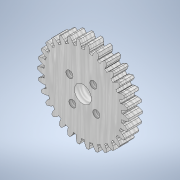
# Autodesk Inventor part: m1歯数30ギア5t
Saved by Autodesk Inventor 2020.2 (Build 242310000, 310)
## iProperties
Created: 2020-02-29
Part Number: m1歯数30ギア5t
Material: アルミニウム 7075
Document SubType Name: Modeling
Designer: aoyam
Density: 2.81 g/cm^3
Appearance: サテン - ブラシ仕上げ 重厚
Author: aoyam
Autodesk Inventor part; units mm, degrees
ref_plane "YZ Plane" through (0, 0, 0) normal (1, 0, 0) x (0, 1, 0)
ref_plane "XZ Plane" through (0, 0, 0) normal (0, 1, 0) x (-1, 0, 0)
ref_plane "XY Plane" through (0, 0, 0) normal (0, 0, 1) x (1, 0, 0)
sketch "スケッチ1" plane through (0, 0, 0) normal (0, 0, 1) x (1, 0, 0)
  arc A0 (3.2208, 16.1154) -> (3.1922, 15.9239) centre (4.5004, 15.8268) ccw
  arc A1 (3.406, 16.7122) -> (3.2208, 16.1154) centre (6.7386, 15.3507) ccw
  arc A2 (3.9698, 17.7851) -> (3.406, 16.7122) centre (9.1484, 14.3793) ccw
  arc A3 (2.1366, 15.9239) -> (2.108, 16.1154) centre (0.8284, 15.8268) ccw
  arc A4 (2.108, 16.1154) -> (1.9228, 16.7122) centre (-1.4098, 15.3507) ccw
  arc A5 (1.9228, 16.7122) -> (1.359, 17.7851) centre (-3.8196, 14.3793) ccw
  arc A6 (3.1793, 15.5788) -> (2.1495, 15.5788) centre (2.6644, 1.8384) ccw
  arc A7 (1.359, 17.7851) -> (0.6257, 17.708) centre (2.6644, 1.8384) ccw
  line L0 (3.1793, 15.5788) -> (3.1922, 15.9239)
  line L1 (2.1495, 15.5788) -> (2.1366, 15.9239)
  arc A8 (0.2403, 15.9191) -> (0.2521, 15.7259) centre (1.5519, 15.9028) ccw
  line L2 (0.3113, 15.3856) -> (0.2521, 15.7259)
  arc A9 (0.2973, 16.5413) -> (0.2403, 15.9191) centre (3.8402, 15.9025) ccw
  arc A10 (0.6257, 17.708) -> (0.2973, 16.5413) centre (6.3993, 15.4534) ccw
  arc A11 (0.3113, 15.3856) -> (-0.696, 15.1715) centre (2.6644, 1.8384) ccw
  line L3 (-0.696, 15.1715) -> (-0.7804, 15.5064)
  arc A12 (-0.7804, 15.5064) -> (-0.8482, 15.6877) centre (-2.0398, 15.1394) ccw
  arc A13 (-1.1534, 16.233) -> (-1.9279, 17.1652) centre (-6.2853, 12.7572) ccw
  arc A14 (-1.9279, 17.1652) -> (-2.6292, 16.9374) centre (2.6644, 1.8384) ccw
  arc A15 (-0.8482, 15.6877) -> (-1.1534, 16.233) centre (-4.1301, 14.2084) ccw
  arc A16 (-2.6343, 15.1074) -> (-2.5825, 14.9209) centre (-1.3479, 15.3642) ccw
  line L4 (-2.4539, 14.6003) -> (-2.5825, 14.9209)
  arc A17 (-2.7078, 15.7279) -> (-2.6343, 15.1074) centre (0.8904, 15.8397) ccw
  arc A18 (-2.6292, 16.9374) -> (-2.7078, 15.7279) centre (3.487, 15.9324) ccw
  arc A19 (-2.4539, 14.6003) -> (-3.3947, 14.1814) centre (2.6644, 1.8384) ccw
  line L5 (-3.3947, 14.1814) -> (-3.5469, 14.4915)
  arc A20 (-3.5469, 14.4915) -> (-3.6508, 14.6548) centre (-4.7024, 13.8707) ccw
  arc A21 (-4.0628, 15.1246) -> (-5.0142, 15.8755) centre (-8.3599, 10.6578) ccw
  arc A22 (-5.0142, 15.8755) -> (-5.6528, 15.5068) centre (2.6644, 1.8384) ccw
  arc A23 (-3.6508, 14.6548) -> (-4.0628, 15.1246) centre (-6.5535, 12.5254) ccw
  arc A24 (-5.2773, 13.7158) -> (-5.1878, 13.5441) centre (-4.0724, 14.2344) ccw
  line L6 (-4.9954, 13.2573) -> (-5.1878, 13.5441)
  arc A25 (-5.4782, 14.3074) -> (-5.2773, 13.7158) centre (-1.9819, 15.1649) ccw
  arc A26 (-5.6528, 15.5068) -> (-5.4782, 14.3074) centre (0.5387, 15.7954) ccw
  arc A27 (-4.9954, 13.2573) -> (-5.8285, 12.652) centre (2.6644, 1.8384) ccw
  line L7 (-5.8285, 12.652) -> (-6.0419, 12.9236)
  arc A28 (-6.0419, 12.9236) -> (-6.1775, 13.0617) centre (-7.0431, 12.0761) ccw
  arc A29 (-6.6781, 13.4356) -> (-7.7649, 13.9723) centre (-9.9526, 8.173) ccw
  arc A30 (-7.7649, 13.9723) -> (-8.3128, 13.4789) centre (2.6644, 1.8384) ccw
  arc A31 (-6.1775, 13.0617) -> (-6.6781, 13.4356) centre (-8.574, 10.3754) ccw
  arc A32 (-7.5732, 11.8051) -> (-7.45, 11.6557) centre (-6.5025, 12.5629) ccw
  line L8 (-7.2021, 11.4152) -> (-7.45, 11.6557)
  arc A33 (-7.8927, 12.342) -> (-7.5732, 11.8051) centre (-4.651, 13.9076) ccw
  arc A34 (-8.3128, 13.4789) -> (-7.8927, 12.342) centre (-2.3167, 15.0485) ccw
  arc A35 (-7.2021, 11.4152) -> (-7.8912, 10.6499) centre (2.6644, 1.8384) ccw
  line L9 (-7.8912, 10.6499) -> (-8.1564, 10.8712)
  arc A36 (-8.1564, 10.8712) -> (-8.3177, 10.9781) centre (-8.9595, 9.8341) ccw
  arc A37 (-8.8852, 11.2398) -> (-10.0597, 11.5388) centre (-10.9939, 5.4114) ccw
  arc A38 (-10.0597, 11.5388) -> (-10.4931, 10.9422) centre (2.6644, 1.8384) ccw
  arc A39 (-8.3177, 10.9781) -> (-8.8852, 11.2398) centre (-10.1034, 7.8522) ccw
  arc A40 (-9.4216, 9.4587) -> (-9.2701, 9.3383) centre (-8.5319, 10.4226) ccw
  line L10 (-8.9777, 9.1545) -> (-9.2701, 9.3383)
  arc A41 (-9.8458, 9.9175) -> (-9.4216, 9.4587) centre (-7.0005, 12.1229) ccw
  arc A42 (-10.4931, 10.9422) -> (-9.8458, 9.9175) centre (-4.9544, 13.7242) ccw
  arc A43 (-8.9777, 9.1545) -> (-9.4925, 8.2627) centre (2.6644, 1.8384) ccw
  line L11 (-9.4925, 8.2627) -> (-9.7979, 8.4241)
  arc A44 (-9.7979, 8.4241) -> (-9.978, 8.4951) centre (-10.3679, 7.2426) ccw
  arc A45 (-10.5874, 8.6331) -> (-11.7985, 8.6813) centre (-11.4383, 2.4936) ccw
  arc A46 (-11.7985, 8.6813) -> (-12.0984, 8.0077) centre (2.6644, 1.8384) ccw
  arc A47 (-9.978, 8.4951) -> (-10.5874, 8.6331) centre (-11.0747, 5.0662) ccw
  arc A48 (-10.7419, 6.7794) -> (-10.5686, 6.6931) centre (-10.072, 7.9072) ccw
  line L12 (-10.2443, 6.5741) -> (-10.5686, 6.6931)
  arc A49 (-11.2522, 7.14) -> (-10.7419, 6.7794) centre (-8.9276, 9.8887) ccw
  arc A50 (-12.0984, 8.0077) -> (-11.2522, 7.14) centre (-7.2591, 11.8804) ccw
  arc A51 (-10.2443, 6.5741) -> (-10.5626, 5.5947) centre (2.6644, 1.8384) ccw
  line L13 (-10.5626, 5.5947) -> (-10.8948, 5.6891)
  arc A52 (-10.8948, 5.6891) -> (-11.0857, 5.7211) centre (-11.2067, 4.4149) ccw
  arc A53 (-11.7105, 5.7294) -> (-12.9052, 5.5247) centre (-11.2664, -0.4529) ccw
  arc A54 (-12.9052, 5.5247) -> (-13.0585, 4.8035) centre (2.6644, 1.8384) ccw
  arc A55 (-11.0857, 5.7211) -> (-11.7105, 5.7294) centre (-11.4456, 2.1392) ccw
  arc A56 (-11.4762, 3.8841) -> (-11.2888, 3.8357) centre (-11.0554, 5.1265) ccw
  line L14 (-10.9469, 3.7868) -> (-11.2888, 3.8357)
  arc A57 (-12.0503, 4.1307) -> (-11.4762, 3.8841) centre (-10.348, 7.3027) ccw
  arc A58 (-13.0585, 4.8035) -> (-12.0503, 4.1307) centre (-9.13, 9.5978) ccw
  arc A59 (-10.9469, 3.7868) -> (-11.0545, 2.7626) centre (2.6644, 1.8384) ccw
  line L15 (-11.0545, 2.7626) -> (-11.3991, 2.7858)
  arc A60 (-11.3991, 2.7858) -> (-11.5925, 2.7775) centre (-11.4392, 1.4747) ccw
  arc A61 (-12.2054, 2.6556) -> (-13.3314, 2.2071) centre (-10.4856, -3.2992) ccw
  arc A62 (-13.3314, 2.2071) -> (-13.3314, 1.4698) centre (2.6644, 1.8384) ccw
  arc A63 (-11.5925, 2.7775) -> (-12.2054, 2.6556) centre (-11.1998, -0.801) ccw
  arc A64 (-11.5925, 0.8994) -> (-11.3991, 0.891) centre (-11.4392, 2.2022) ccw
  line L16 (-11.0545, 0.9142) -> (-11.3991, 0.891)
  arc A65 (-12.2054, 1.0212) -> (-11.5925, 0.8994) centre (-11.1998, 4.4779) ccw
  arc A66 (-13.3314, 1.4698) -> (-12.2054, 1.0212) centre (-10.4856, 6.976) ccw
  arc A67 (-11.0545, 0.9142) -> (-10.9469, -0.1099) centre (2.6644, 1.8384) ccw
  line L17 (-10.9469, -0.1099) -> (-11.2888, -0.1588)
  arc A68 (-11.2888, -0.1588) -> (-11.4762, -0.2072) centre (-11.0554, -1.4497) ccw
  arc A69 (-12.0503, -0.4538) -> (-13.0585, -1.1267) centre (-9.13, -5.9209) ccw
  arc A70 (-13.0585, -1.1267) -> (-12.9052, -1.8479) centre (2.6644, 1.8384) ccw
  arc A71 (-11.4762, -0.2072) -> (-12.0503, -0.4538) centre (-10.348, -3.6259) ccw
  arc A72 (-11.0857, -2.0443) -> (-10.8948, -2.0122) centre (-11.2067, -0.7381) ccw
  line L18 (-10.5626, -1.9179) -> (-10.8948, -2.0122)
  arc A73 (-11.7105, -2.0525) -> (-11.0857, -2.0443) centre (-11.4456, 1.5377) ccw
  arc A74 (-12.9052, -1.8479) -> (-11.7105, -2.0525) centre (-11.2664, 4.1297) ccw
  arc A75 (-10.5626, -1.9179) -> (-10.2443, -2.8973) centre (2.6644, 1.8384) ccw
  line L19 (-10.2443, -2.8973) -> (-10.5686, -3.0162)
  arc A76 (-10.5686, -3.0162) -> (-10.7419, -3.1025) centre (-10.072, -4.2303) ccw
  arc A77 (-11.2522, -3.4631) -> (-12.0984, -4.3308) centre (-7.2591, -8.2036) ccw
  arc A78 (-12.0984, -4.3308) -> (-11.7985, -5.0044) centre (2.6644, 1.8384) ccw
  arc A79 (-10.7419, -3.1025) -> (-11.2522, -3.4631) centre (-8.9276, -6.2119) ccw
  arc A80 (-9.978, -4.8182) -> (-9.7979, -4.7472) centre (-10.3679, -3.5657) ccw
  line L20 (-9.4925, -4.5858) -> (-9.7979, -4.7472)
  arc A81 (-10.5874, -4.9562) -> (-9.978, -4.8182) centre (-11.0747, -1.3894) ccw
  arc A82 (-11.7985, -5.0044) -> (-10.5874, -4.9562) centre (-11.4383, 1.1833) ccw
  arc A83 (-9.4925, -4.5858) -> (-8.9777, -5.4777) centre (2.6644, 1.8384) ccw
  line L21 (-8.9777, -5.4777) -> (-9.2701, -5.6614)
  arc A84 (-9.2701, -5.6614) -> (-9.4216, -5.7819) centre (-8.5319, -6.7458) ccw
  arc A85 (-9.8458, -6.2407) -> (-10.4931, -7.2654) centre (-4.9544, -10.0473) ccw
  arc A86 (-10.4931, -7.2654) -> (-10.0597, -7.8619) centre (2.6644, 1.8384) ccw
  arc A87 (-9.4216, -5.7819) -> (-9.8458, -6.2407) centre (-7.0005, -8.4461) ccw
  arc A88 (-8.3177, -7.3013) -> (-8.1564, -7.1944) centre (-8.9595, -6.1572) ccw
  line L22 (-7.8912, -6.973) -> (-8.1564, -7.1944)
  arc A89 (-8.8852, -7.5629) -> (-8.3177, -7.3013) centre (-10.1034, -4.1754) ccw
  arc A90 (-10.0597, -7.8619) -> (-8.8852, -7.5629) centre (-10.9939, -1.7345) ccw
  arc A91 (-7.8912, -6.973) -> (-7.2021, -7.7383) centre (2.6644, 1.8384) ccw
  line L23 (-7.2021, -7.7383) -> (-7.45, -7.9789)
  arc A92 (-7.45, -7.9789) -> (-7.5732, -8.1282) centre (-6.5025, -8.886) ccw
  arc A93 (-7.8927, -8.6651) -> (-8.3128, -9.802) centre (-2.3167, -11.3716) ccw
  arc A94 (-8.3128, -9.802) -> (-7.7649, -10.2954) centre (2.6644, 1.8384) ccw
  arc A95 (-7.5732, -8.1282) -> (-7.8927, -8.6651) centre (-4.651, -10.2308) ccw
  arc A96 (-6.1775, -9.3849) -> (-6.0419, -9.2467) centre (-7.0431, -8.3992) ccw
  line L24 (-5.8285, -8.9751) -> (-6.0419, -9.2467)
  arc A97 (-6.6781, -9.7588) -> (-6.1775, -9.3849) centre (-8.574, -6.6985) ccw
  arc A98 (-7.7649, -10.2954) -> (-6.6781, -9.7588) centre (-9.9526, -4.4962) ccw
  arc A99 (-5.8285, -8.9751) -> (-4.9954, -9.5804) centre (2.6644, 1.8384) ccw
  line L25 (-4.9954, -9.5804) -> (-5.1878, -9.8672)
  arc A100 (-5.1878, -9.8672) -> (-5.2773, -10.0389) centre (-4.0724, -10.5575) ccw
  arc A101 (-5.4782, -10.6306) -> (-5.6528, -11.83) centre (0.5387, -12.1186) ccw
  arc A102 (-5.6528, -11.83) -> (-5.0142, -12.1986) centre (2.6644, 1.8384) ccw
  arc A103 (-5.2773, -10.0389) -> (-5.4782, -10.6306) centre (-1.9819, -11.488) ccw
  arc A104 (-3.6508, -10.9779) -> (-3.5469, -10.8146) centre (-4.7024, -10.1938) ccw
  line L26 (-3.3947, -10.5046) -> (-3.5469, -10.8146)
  arc A105 (-4.0628, -11.4478) -> (-3.6508, -10.9779) centre (-6.5535, -8.8486) ccw
  arc A106 (-5.0142, -12.1986) -> (-4.0628, -11.4478) centre (-8.3599, -6.981) ccw
  arc A107 (-3.3947, -10.5046) -> (-2.4539, -10.9234) centre (2.6644, 1.8384) ccw
  line L27 (-2.4539, -10.9234) -> (-2.5825, -11.244)
  arc A108 (-2.5825, -11.244) -> (-2.6343, -11.4305) centre (-1.3479, -11.6873) ccw
  arc A109 (-2.7078, -12.051) -> (-2.6292, -13.2605) centre (3.487, -12.2555) ccw
  arc A110 (-2.6292, -13.2605) -> (-1.9279, -13.4884) centre (2.6644, 1.8384) ccw
  arc A111 (-2.6343, -11.4305) -> (-2.7078, -12.051) centre (0.8904, -12.1628) ccw
  arc A112 (-0.8482, -12.0109) -> (-0.7804, -11.8295) centre (-2.0398, -11.4625) ccw
  line L28 (-0.696, -11.4946) -> (-0.7804, -11.8295)
  arc A113 (-1.1534, -12.5561) -> (-0.8482, -12.0109) centre (-4.1301, -10.5315) ccw
  arc A114 (-1.9279, -13.4884) -> (-1.1534, -12.5561) centre (-6.2853, -9.0803) ccw
  arc A115 (-0.696, -11.4946) -> (0.3113, -11.7087) centre (2.6644, 1.8384) ccw
  line L29 (0.3113, -11.7087) -> (0.2521, -12.049)
  arc A116 (0.2521, -12.049) -> (0.2403, -12.2422) centre (1.5519, -12.226) ccw
  arc A117 (0.2973, -12.8645) -> (0.6257, -14.0312) centre (6.3993, -11.7765) ccw
  arc A118 (0.6257, -14.0312) -> (1.359, -14.1082) centre (2.6644, 1.8384) ccw
  arc A119 (0.2403, -12.2422) -> (0.2973, -12.8645) centre (3.8402, -12.2257) ccw
  arc A120 (2.108, -12.4385) -> (2.1366, -12.2471) centre (0.8284, -12.1499) ccw
  line L30 (2.1495, -11.9019) -> (2.1366, -12.2471)
  arc A121 (1.9228, -13.0353) -> (2.108, -12.4385) centre (-1.4098, -11.6739) ccw
  arc A122 (1.359, -14.1082) -> (1.9228, -13.0353) centre (-3.8196, -10.7025) ccw
  arc A123 (2.1495, -11.9019) -> (3.1793, -11.9019) centre (2.6644, 1.8384) ccw
  line L31 (3.1793, -11.9019) -> (3.1922, -12.2471)
  arc A124 (3.1922, -12.2471) -> (3.2208, -12.4385) centre (4.5004, -12.1499) ccw
  arc A125 (3.406, -13.0353) -> (3.9698, -14.1082) centre (9.1484, -10.7025) ccw
  arc A126 (3.9698, -14.1082) -> (4.7031, -14.0312) centre (2.6644, 1.8384) ccw
  arc A127 (3.2208, -12.4385) -> (3.406, -13.0353) centre (6.7386, -11.6739) ccw
  arc A128 (5.0885, -12.2422) -> (5.0766, -12.049) centre (3.7769, -12.226) ccw
  line L32 (5.0175, -11.7087) -> (5.0766, -12.049)
  arc A129 (5.0314, -12.8645) -> (5.0885, -12.2422) centre (1.4886, -12.2257) ccw
  arc A130 (4.7031, -14.0312) -> (5.0314, -12.8645) centre (-1.0705, -11.7765) ccw
  arc A131 (5.0175, -11.7087) -> (6.0248, -11.4946) centre (2.6644, 1.8384) ccw
  line L33 (6.0248, -11.4946) -> (6.1092, -11.8295)
  arc A132 (6.1092, -11.8295) -> (6.177, -12.0109) centre (7.3686, -11.4625) ccw
  arc A133 (6.4822, -12.5561) -> (7.2567, -13.4884) centre (11.6141, -9.0803) ccw
  arc A134 (7.2567, -13.4884) -> (7.958, -13.2605) centre (2.6644, 1.8384) ccw
  arc A135 (6.177, -12.0109) -> (6.4822, -12.5561) centre (9.4589, -10.5315) ccw
  arc A136 (7.9631, -11.4305) -> (7.9113, -11.244) centre (6.6767, -11.6873) ccw
  line L34 (7.7827, -10.9234) -> (7.9113, -11.244)
  arc A137 (8.0366, -12.051) -> (7.9631, -11.4305) centre (4.4384, -12.1628) ccw
  arc A138 (7.958, -13.2605) -> (8.0366, -12.051) centre (1.8418, -12.2555) ccw
  arc A139 (7.7827, -10.9234) -> (8.7235, -10.5046) centre (2.6644, 1.8384) ccw
  line L35 (8.7235, -10.5046) -> (8.8757, -10.8146)
  arc A140 (8.8757, -10.8146) -> (8.9796, -10.9779) centre (10.0312, -10.1938) ccw
  arc A141 (9.3916, -11.4478) -> (10.343, -12.1986) centre (13.6887, -6.981) ccw
  arc A142 (10.343, -12.1986) -> (10.9815, -11.83) centre (2.6644, 1.8384) ccw
  arc A143 (8.9796, -10.9779) -> (9.3916, -11.4478) centre (11.8823, -8.8486) ccw
  arc A144 (10.6061, -10.0389) -> (10.5166, -9.8672) centre (9.4012, -10.5575) ccw
  line L36 (10.3242, -9.5804) -> (10.5166, -9.8672)
  arc A145 (10.807, -10.6306) -> (10.6061, -10.0389) centre (7.3106, -11.488) ccw
  arc A146 (10.9815, -11.83) -> (10.807, -10.6306) centre (4.7901, -12.1186) ccw
  arc A147 (10.3242, -9.5804) -> (11.1573, -8.9751) centre (2.6644, 1.8384) ccw
  line L37 (11.1573, -8.9751) -> (11.3707, -9.2467)
  arc A148 (11.3707, -9.2467) -> (11.5063, -9.3849) centre (12.3719, -8.3992) ccw
  arc A149 (12.0069, -9.7588) -> (13.0937, -10.2954) centre (15.2814, -4.4962) ccw
  arc A150 (13.0937, -10.2954) -> (13.6416, -9.802) centre (2.6644, 1.8384) ccw
  arc A151 (11.5063, -9.3849) -> (12.0069, -9.7588) centre (13.9028, -6.6985) ccw
  arc A152 (12.902, -8.1282) -> (12.7788, -7.9789) centre (11.8312, -8.886) ccw
  line L38 (12.5309, -7.7383) -> (12.7788, -7.9789)
  arc A153 (13.2215, -8.6651) -> (12.902, -8.1282) centre (9.9798, -10.2308) ccw
  arc A154 (13.6416, -9.802) -> (13.2215, -8.6651) centre (7.6455, -11.3716) ccw
  arc A155 (12.5309, -7.7383) -> (13.22, -6.973) centre (2.6644, 1.8384) ccw
  line L39 (13.22, -6.973) -> (13.4851, -7.1944)
  arc A156 (13.4851, -7.1944) -> (13.6465, -7.3013) centre (14.2883, -6.1572) ccw
  arc A157 (14.214, -7.5629) -> (15.3885, -7.8619) centre (16.3227, -1.7345) ccw
  arc A158 (15.3885, -7.8619) -> (15.8219, -7.2654) centre (2.6644, 1.8384) ccw
  arc A159 (13.6465, -7.3013) -> (14.214, -7.5629) centre (15.4322, -4.1754) ccw
  arc A160 (14.7504, -5.7819) -> (14.5989, -5.6614) centre (13.8607, -6.7458) ccw
  line L40 (14.3064, -5.4777) -> (14.5989, -5.6614)
  arc A161 (15.1746, -6.2407) -> (14.7504, -5.7819) centre (12.3293, -8.4461) ccw
  arc A162 (15.8219, -7.2654) -> (15.1746, -6.2407) centre (10.2831, -10.0473) ccw
  arc A163 (14.3064, -5.4777) -> (14.8213, -4.5858) centre (2.6644, 1.8384) ccw
  line L41 (14.8213, -4.5858) -> (15.1267, -4.7472)
  arc A164 (15.1267, -4.7472) -> (15.3068, -4.8182) centre (15.6966, -3.5657) ccw
  arc A165 (15.9162, -4.9562) -> (17.1273, -5.0044) centre (16.7671, 1.1833) ccw
  arc A166 (17.1273, -5.0044) -> (17.4272, -4.3308) centre (2.6644, 1.8384) ccw
  arc A167 (15.3068, -4.8182) -> (15.9162, -4.9562) centre (16.4035, -1.3894) ccw
  arc A168 (16.0707, -3.1025) -> (15.8974, -3.0162) centre (15.4007, -4.2303) ccw
  line L42 (15.5731, -2.8973) -> (15.8974, -3.0162)
  arc A169 (16.581, -3.4631) -> (16.0707, -3.1025) centre (14.2564, -6.2119) ccw
  arc A170 (17.4272, -4.3308) -> (16.581, -3.4631) centre (12.5878, -8.2036) ccw
  arc A171 (15.5731, -2.8973) -> (15.8914, -1.9179) centre (2.6644, 1.8384) ccw
  line L43 (15.8914, -1.9179) -> (16.2236, -2.0122)
  arc A172 (16.2236, -2.0122) -> (16.4145, -2.0443) centre (16.5355, -0.7381) ccw
  arc A173 (17.0393, -2.0525) -> (18.234, -1.8479) centre (16.5952, 4.1297) ccw
  arc A174 (18.234, -1.8479) -> (18.3873, -1.1267) centre (2.6644, 1.8384) ccw
  arc A175 (16.4145, -2.0443) -> (17.0393, -2.0525) centre (16.7744, 1.5377) ccw
  arc A176 (16.805, -0.2072) -> (16.6176, -0.1588) centre (16.3842, -1.4497) ccw
  line L44 (16.2757, -0.1099) -> (16.6176, -0.1588)
  arc A177 (17.3791, -0.4538) -> (16.805, -0.2072) centre (15.6768, -3.6259) ccw
  arc A178 (18.3873, -1.1267) -> (17.3791, -0.4538) centre (14.4588, -5.9209) ccw
  arc A179 (16.2757, -0.1099) -> (16.3833, 0.9142) centre (2.6644, 1.8384) ccw
  line L45 (16.3833, 0.9142) -> (16.7279, 0.891)
  arc A180 (16.7279, 0.891) -> (16.9213, 0.8994) centre (16.768, 2.2022) ccw
  arc A181 (17.5342, 1.0212) -> (18.6601, 1.4698) centre (15.8144, 6.976) ccw
  arc A182 (18.6601, 1.4698) -> (18.6601, 2.2071) centre (2.6644, 1.8384) ccw
  arc A183 (16.9213, 0.8994) -> (17.5342, 1.0212) centre (16.5286, 4.4779) ccw
  arc A184 (16.9213, 2.7775) -> (16.7279, 2.7858) centre (16.768, 1.4747) ccw
  line L46 (16.3833, 2.7626) -> (16.7279, 2.7858)
  arc A185 (17.5342, 2.6556) -> (16.9213, 2.7775) centre (16.5286, -0.801) ccw
  arc A186 (18.6601, 2.2071) -> (17.5342, 2.6556) centre (15.8144, -3.2992) ccw
  arc A187 (16.3833, 2.7626) -> (16.2757, 3.7868) centre (2.6644, 1.8384) ccw
  line L47 (16.2757, 3.7868) -> (16.6176, 3.8357)
  arc A188 (16.6176, 3.8357) -> (16.805, 3.8841) centre (16.3842, 5.1265) ccw
  arc A189 (17.3791, 4.1307) -> (18.3873, 4.8035) centre (14.4588, 9.5978) ccw
  arc A190 (18.3873, 4.8035) -> (18.234, 5.5247) centre (2.6644, 1.8384) ccw
  arc A191 (16.805, 3.8841) -> (17.3791, 4.1307) centre (15.6768, 7.3027) ccw
  arc A192 (16.4145, 5.7211) -> (16.2236, 5.6891) centre (16.5355, 4.4149) ccw
  line L48 (15.8914, 5.5947) -> (16.2236, 5.6891)
  arc A193 (17.0393, 5.7294) -> (16.4145, 5.7211) centre (16.7744, 2.1392) ccw
  arc A194 (18.234, 5.5247) -> (17.0393, 5.7294) centre (16.5952, -0.4529) ccw
  arc A195 (15.8914, 5.5947) -> (15.5731, 6.5741) centre (2.6644, 1.8384) ccw
  line L49 (15.5731, 6.5741) -> (15.8974, 6.6931)
  arc A196 (15.8974, 6.6931) -> (16.0707, 6.7794) centre (15.4007, 7.9072) ccw
  arc A197 (16.581, 7.14) -> (17.4272, 8.0077) centre (12.5878, 11.8804) ccw
  arc A198 (17.4272, 8.0077) -> (17.1273, 8.6813) centre (2.6644, 1.8384) ccw
  arc A199 (16.0707, 6.7794) -> (16.581, 7.14) centre (14.2564, 9.8887) ccw
  arc A200 (15.3068, 8.4951) -> (15.1267, 8.4241) centre (15.6966, 7.2426) ccw
  line L50 (14.8213, 8.2627) -> (15.1267, 8.4241)
  arc A201 (15.9162, 8.6331) -> (15.3068, 8.4951) centre (16.4035, 5.0662) ccw
  arc A202 (17.1273, 8.6813) -> (15.9162, 8.6331) centre (16.7671, 2.4936) ccw
  arc A203 (14.8213, 8.2627) -> (14.3064, 9.1545) centre (2.6644, 1.8384) ccw
  line L51 (14.3064, 9.1545) -> (14.5989, 9.3383)
  arc A204 (14.5989, 9.3383) -> (14.7504, 9.4587) centre (13.8607, 10.4226) ccw
  arc A205 (15.1746, 9.9175) -> (15.8219, 10.9422) centre (10.2831, 13.7242) ccw
  arc A206 (15.8219, 10.9422) -> (15.3885, 11.5388) centre (2.6644, 1.8384) ccw
  arc A207 (14.7504, 9.4587) -> (15.1746, 9.9175) centre (12.3293, 12.1229) ccw
  arc A208 (13.6465, 10.9781) -> (13.4851, 10.8712) centre (14.2883, 9.8341) ccw
  line L52 (13.22, 10.6499) -> (13.4851, 10.8712)
  arc A209 (14.214, 11.2398) -> (13.6465, 10.9781) centre (15.4322, 7.8522) ccw
  arc A210 (15.3885, 11.5388) -> (14.214, 11.2398) centre (16.3227, 5.4114) ccw
  arc A211 (13.22, 10.6499) -> (12.5309, 11.4152) centre (2.6644, 1.8384) ccw
  line L53 (12.5309, 11.4152) -> (12.7788, 11.6557)
  arc A212 (12.7788, 11.6557) -> (12.902, 11.8051) centre (11.8312, 12.5629) ccw
  arc A213 (13.2215, 12.342) -> (13.6416, 13.4789) centre (7.6455, 15.0485) ccw
  arc A214 (13.6416, 13.4789) -> (13.0937, 13.9723) centre (2.6644, 1.8384) ccw
  arc A215 (12.902, 11.8051) -> (13.2215, 12.342) centre (9.9798, 13.9076) ccw
  arc A216 (11.5063, 13.0617) -> (11.3707, 12.9236) centre (12.3719, 12.0761) ccw
  line L54 (11.1573, 12.652) -> (11.3707, 12.9236)
  arc A217 (12.0069, 13.4356) -> (11.5063, 13.0617) centre (13.9028, 10.3754) ccw
  arc A218 (13.0937, 13.9723) -> (12.0069, 13.4356) centre (15.2814, 8.173) ccw
  arc A219 (11.1573, 12.652) -> (10.3242, 13.2573) centre (2.6644, 1.8384) ccw
  line L55 (10.3242, 13.2573) -> (10.5166, 13.5441)
  arc A220 (10.5166, 13.5441) -> (10.6061, 13.7158) centre (9.4012, 14.2344) ccw
  arc A221 (10.807, 14.3074) -> (10.9815, 15.5068) centre (4.7901, 15.7954) ccw
  arc A222 (10.9815, 15.5068) -> (10.343, 15.8755) centre (2.6644, 1.8384) ccw
  arc A223 (10.6061, 13.7158) -> (10.807, 14.3074) centre (7.3106, 15.1649) ccw
  arc A224 (8.9796, 14.6548) -> (8.8757, 14.4915) centre (10.0312, 13.8707) ccw
  line L56 (8.7235, 14.1814) -> (8.8757, 14.4915)
  arc A225 (9.3916, 15.1246) -> (8.9796, 14.6548) centre (11.8823, 12.5254) ccw
  arc A226 (10.343, 15.8755) -> (9.3916, 15.1246) centre (13.6887, 10.6578) ccw
  arc A227 (8.7235, 14.1814) -> (7.7827, 14.6003) centre (2.6644, 1.8384) ccw
  line L57 (7.7827, 14.6003) -> (7.9113, 14.9209)
  arc A228 (7.9113, 14.9209) -> (7.9631, 15.1074) centre (6.6767, 15.3642) ccw
  arc A229 (8.0366, 15.7279) -> (7.958, 16.9374) centre (1.8418, 15.9324) ccw
  arc A230 (7.958, 16.9374) -> (7.2567, 17.1652) centre (2.6644, 1.8384) ccw
  arc A231 (7.9631, 15.1074) -> (8.0366, 15.7279) centre (4.4384, 15.8397) ccw
  arc A232 (6.177, 15.6877) -> (6.1092, 15.5064) centre (7.3686, 15.1394) ccw
  line L58 (6.0248, 15.1715) -> (6.1092, 15.5064)
  arc A233 (6.4822, 16.233) -> (6.177, 15.6877) centre (9.4589, 14.2084) ccw
  arc A234 (7.2567, 17.1652) -> (6.4822, 16.233) centre (11.6141, 12.7572) ccw
  arc A235 (6.0248, 15.1715) -> (5.0175, 15.3856) centre (2.6644, 1.8384) ccw
  line L59 (5.0175, 15.3856) -> (5.0766, 15.7259)
  arc A236 (5.0766, 15.7259) -> (5.0885, 15.9191) centre (3.7769, 15.9028) ccw
  arc A237 (5.0314, 16.5413) -> (4.7031, 17.708) centre (-1.0705, 15.4534) ccw
  arc A238 (4.7031, 17.708) -> (3.9698, 17.7851) centre (2.6644, 1.8384) ccw
  arc A239 (5.0885, 15.9191) -> (5.0314, 16.5413) centre (1.4886, 15.9025) ccw
  circle A240 centre (2.6644, 1.8384) radius 2.99
  point P0 (0, 0)
  point P1 (-0.8482, 15.6877)
  point P2 (-1.1534, 16.233)
  point P3 (-1.9279, 17.1652)
  point P4 (-2.6292, 16.9374)
  point P5 (-2.7078, 15.7279)
  point P6 (-2.6343, 15.1074)
  point P7 (-2.5825, 14.9209)
  point P8 (-2.4539, 14.6003)
  point P9 (-3.3947, 14.1814)
  point P10 (-3.6508, 14.6548)
  point P11 (-4.0628, 15.1246)
  point P12 (-5.0142, 15.8755)
  point P13 (-5.6528, 15.5068)
  point P14 (-5.4782, 14.3074)
  point P15 (-5.2773, 13.7158)
  point P16 (-4.9954, 13.2573)
  point P17 (-5.8285, 12.652)
  point P18 (-6.0419, 12.9236)
  point P19 (-6.1775, 13.0617)
  point P20 (-6.6781, 13.4356)
  point P21 (-7.7649, 13.9723)
  point P22 (-8.3128, 13.4789)
  point P23 (-7.8927, 12.342)
  point P24 (-7.5732, 11.8051)
  point P25 (-8.3177, 10.9781)
  point P26 (-8.8852, 11.2398)
  point P27 (-10.0597, 11.5388)
  point P28 (-10.4931, 10.9422)
  point P29 (-9.8458, 9.9175)
  point P30 (-9.4216, 9.4587)
  point P31 (-9.2701, 9.3383)
  point P32 (-9.978, 8.4951)
  point P33 (-10.5874, 8.6331)
  point P34 (-11.7985, 8.6813)
  point P35 (-12.0984, 8.0077)
  point P36 (-11.2522, 7.14)
  point P37 (-10.7419, 6.7794)
  point P38 (-10.8948, 5.6891)
  point P39 (-11.0857, 5.7211)
  point P40 (-11.7105, 5.7294)
  point P41 (-12.9052, 5.5247)
  point P42 (-13.0585, 4.8035)
  point P43 (-12.0503, 4.1307)
  point P44 (-11.4762, 3.8841)
  point P45 (-11.5925, 2.7775)
  point P46 (-12.2054, 2.6556)
  point P47 (-13.3314, 2.2071)
  point P48 (-13.3314, 1.4698)
  point P49 (-12.2054, 1.0212)
  point P50 (-11.5925, 0.8994)
  point P51 (-11.3991, 0.891)
  point P52 (-11.0545, 0.9142)
  point P53 (-11.4762, -0.2072)
  point P54 (-12.0503, -0.4538)
  point P55 (-13.0585, -1.1267)
  point P56 (-12.9052, -1.8479)
  point P57 (-11.7105, -2.0525)
  point P58 (-11.0857, -2.0443)
  point P59 (-10.8948, -2.0122)
  point P60 (-10.5626, -1.9179)
  point P61 (-10.2443, -2.8973)
  point P62 (-10.7419, -3.1025)
  point P63 (-11.2522, -3.4631)
  point P64 (-12.0984, -4.3308)
  point P65 (-11.7985, -5.0044)
  point P66 (-10.5874, -4.9562)
  point P67 (-9.978, -4.8182)
  point P68 (-9.7979, -4.7472)
  point P69 (-9.4216, -5.7819)
  point P70 (-9.8458, -6.2407)
  point P71 (-10.4931, -7.2654)
  point P72 (-10.0597, -7.8619)
  point P73 (-8.8852, -7.5629)
  point P74 (-8.3177, -7.3013)
  point P75 (-8.1564, -7.1944)
  point P76 (-7.8912, -6.973)
  point P77 (-7.2021, -7.7383)
  point P78 (-7.5732, -8.1282)
  point P79 (-7.8927, -8.6651)
  point P80 (-8.3128, -9.802)
  point P81 (-7.7649, -10.2954)
  point P82 (-6.6781, -9.7588)
  point P83 (-6.1775, -9.3849)
  point P84 (-4.9954, -9.5804)
  point P85 (-5.2773, -10.0389)
  point P86 (-5.4782, -10.6306)
  point P87 (-5.6528, -11.83)
  point P88 (-5.0142, -12.1986)
  point P89 (-4.0628, -11.4478)
  point P90 (-3.6508, -10.9779)
  point P91 (-2.6343, -11.4305)
  point P92 (-2.7078, -12.051)
  point P93 (-2.6292, -13.2605)
  point P94 (-1.9279, -13.4884)
  point P95 (-1.1534, -12.5561)
  point P96 (-0.8482, -12.0109)
  point P97 (-0.696, -11.4946)
  point P98 (0.3113, -11.7087)
  point P99 (0.2521, -12.049)
  point P100 (0.2403, -12.2422)
  point P101 (0.2973, -12.8645)
  point P102 (0.6257, -14.0312)
  point P103 (1.359, -14.1082)
  point P104 (1.9228, -13.0353)
  point P105 (2.108, -12.4385)
  point P106 (3.2208, -12.4385)
  point P107 (3.406, -13.0353)
  point P108 (3.9698, -14.1082)
  point P109 (4.7031, -14.0312)
  point P110 (5.0314, -12.8645)
  point P111 (5.0885, -12.2422)
  point P112 (6.0248, -11.4946)
  point P113 (6.1092, -11.8295)
  point P114 (6.177, -12.0109)
  point P115 (6.4822, -12.5561)
  point P116 (7.2567, -13.4884)
  point P117 (7.958, -13.2605)
  point P118 (8.0366, -12.051)
  point P119 (7.9631, -11.4305)
  point P120 (7.7827, -10.9234)
  point P121 (8.7235, -10.5046)
  point P122 (8.9796, -10.9779)
  point P123 (9.3916, -11.4478)
  point P124 (10.343, -12.1986)
  point P125 (10.9815, -11.83)
  point P126 (10.807, -10.6306)
  point P127 (10.6061, -10.0389)
  point P128 (10.5166, -9.8672)
  point P129 (10.3242, -9.5804)
  point P130 (11.1573, -8.9751)
  point P131 (11.3707, -9.2467)
  point P132 (11.5063, -9.3849)
  point P133 (12.0069, -9.7588)
  point P134 (13.0937, -10.2954)
  point P135 (13.6416, -9.802)
  point P136 (13.2215, -8.6651)
  point P137 (12.902, -8.1282)
  point P138 (12.5309, -7.7383)
  point P139 (13.6465, -7.3013)
  point P140 (14.214, -7.5629)
  point P141 (15.3885, -7.8619)
  point P142 (15.8219, -7.2654)
  point P143 (15.1746, -6.2407)
  point P144 (14.7504, -5.7819)
  point P145 (14.3064, -5.4777)
  point P146 (14.8213, -4.5858)
  point P147 (15.1267, -4.7472)
  point P148 (15.3068, -4.8182)
  point P149 (15.9162, -4.9562)
  point P150 (17.1273, -5.0044)
  point P151 (17.4272, -4.3308)
  point P152 (16.581, -3.4631)
  point P153 (16.0707, -3.1025)
  point P154 (16.4145, -2.0443)
  point P155 (17.0393, -2.0525)
  point P156 (18.234, -1.8479)
  point P157 (18.3873, -1.1267)
  point P158 (17.3791, -0.4538)
  point P159 (16.805, -0.2072)
  point P160 (16.9213, 0.8994)
  point P161 (17.5342, 1.0212)
  point P162 (18.6601, 1.4698)
  point P163 (18.6601, 2.2071)
  point P164 (17.5342, 2.6556)
  point P165 (16.9213, 2.7775)
  point P166 (16.6176, 3.8357)
  point P167 (16.805, 3.8841)
  point P168 (17.3791, 4.1307)
  point P169 (18.3873, 4.8035)
  point P170 (18.234, 5.5247)
  point P171 (17.0393, 5.7294)
  point P172 (16.4145, 5.7211)
  point P173 (15.5731, 6.5741)
  point P174 (15.8974, 6.6931)
  point P175 (16.0707, 6.7794)
  point P176 (16.581, 7.14)
  point P177 (17.4272, 8.0077)
  point P178 (17.1273, 8.6813)
  point P179 (15.9162, 8.6331)
  point P180 (15.3068, 8.4951)
  point P181 (14.8213, 8.2627)
  point P182 (14.3064, 9.1545)
  point P183 (14.5989, 9.3383)
  point P184 (14.7504, 9.4587)
  point P185 (15.1746, 9.9175)
  point P186 (15.8219, 10.9422)
  point P187 (15.3885, 11.5388)
  point P188 (14.214, 11.2398)
  point P189 (13.6465, 10.9781)
  point P190 (13.22, 10.6499)
  point P191 (12.7788, 11.6557)
  point P192 (12.902, 11.8051)
  point P193 (13.2215, 12.342)
  point P194 (13.6416, 13.4789)
  point P195 (13.0937, 13.9723)
  point P196 (12.0069, 13.4356)
  point P197 (11.5063, 13.0617)
  point P198 (11.1573, 12.652)
  point P199 (10.3242, 13.2573)
  dimension "d2" = 360
  dimension "d4" = 5.98
  constraints: 480 point on circle, 241 centre point, 120 end point, 2 coincident, 1139 other
  measures "d4" diameter of A240
extrude "押し出し1" add sketch "スケッチ1" along normal blind 5
sketch "スケッチ2" plane through (0, 0, 5) normal (0, 0, 1) x (1, 0, 0)
  circle A0 centre (2.6644, 1.8384) radius 2.99 projected
  circle A1 centre (-2.0687, 5.5259) radius 1.25
  circle A2 centre (-1.0231, -2.8947) radius 1.25
  circle A3 centre (7.3975, -1.849) radius 1.25
  circle A4 centre (6.3519, 6.5716) radius 1.25
  point P0 (0, 0)
  dimension "d7" = 2.5
  dimension "d8" = 6
  dimension "d11" = 360
  constraints: 4 centre point, 9 other
  measures "d7" diameter of A1
  measures "d8" distance of A0.centre A1.centre
extrude "押し出し2" cut sketch "スケッチ2" against normal blind 6 contours A1 | A2 | A3 | A4
thread "ねじ1" size "M3x0.5" class "6H" standard "ANSI Metric M Profile" full length
thread "ねじ2" size "M3x0.5" class "6H" standard "ANSI Metric M Profile" full length
thread "ねじ3" size "M3x0.5" class "6H" standard "ANSI Metric M Profile" full length
thread "ねじ4" size "M3x0.5" class "6H" standard "ANSI Metric M Profile" full length
